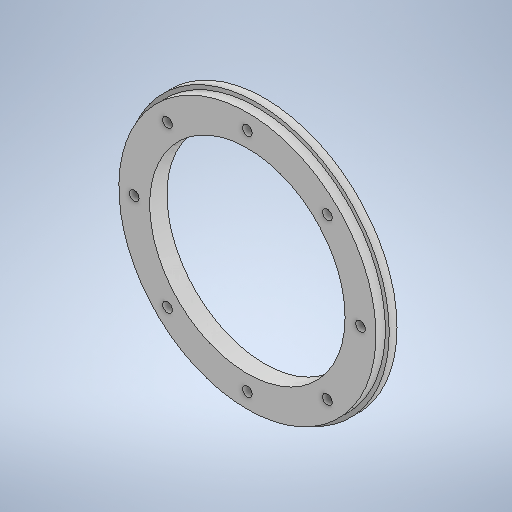
# Autodesk Inventor part: ДМФ 01 31.1 Барабан Опорное кольцо НОС
Saved by Autodesk Inventor 2025 (Build 290162010, 162A)
## iProperties
Created: 2024-04-28
Part Number: ДМФ 01 31.1 Барабан Опорное кольцо НОС
Material: Generic
Document SubType Name: Sheet Metal
Designer: pokla
Density: 1 g/cm^3
Appearance: Default
Stock Number: Опорное_Кольцо_Нос
Sheet Metal Rule: Default
Flat Pattern Width: 33.9 cm
Flat Pattern Length: 33.9 cm
Flat Pattern Area: 1149.21 cm^2
Sheet Metal Width: 339,000 mm
Sheet Metal Length: 339,000 mm
Sheet Metal Area: 114921,000 mm^2
Author: pokla
Autodesk Inventor part; units mm, degrees
ref_plane "YZ Plane" through (0, 0, 0) normal (1, 0, 0) x (0, 1, 0)
ref_plane "XZ Plane" through (0, 0, 0) normal (0, 1, 0) x (-1, 0, 0)
ref_plane "XY Plane" through (0, 0, 0) normal (0, 0, 1) x (1, 0, 0)
sketch "Sketch1" plane through (0, 0, 0) normal (0, 0, 1) x (1, 0, 0)
  circle A0 centre (0, 0) radius 125
  circle A1 centre (0, 0) radius 164.5
  dimension "d0" = 39.5
  dimension "d1" = 250
  constraints: 2 centre point, 1 coincident
  measures "d0" radial gap between concentric circles of A0 A1
  measures "d1" diameter of A0
extrude "Extrusion1" add sketch "Sketch1" along normal blind 41
sketch "Sketch2" plane through (0, 0, 41) normal (0, 0, 1) x (1, 0, 0)
  circle A0 centre (0, 0) radius 164.5 construction
  circle A1 centre (0, 0) radius 125 construction
  line L0 (0, 164.5) -> (0, 125) construction
  circle A2 centre (0, 144.75) radius 6.25
  dimension "d4" = 12.5
  constraints: 3 vertical alignment, 2 end point, 1 centre point, 1 coincident, 1 midpoint, 1 vertical, 2 other
  measures "d4" diameter of A2
extrude "Extrusion2" cut sketch "Sketch2" against normal through all
sketch "Sketch3" plane through (0, 0, 41) normal (0, 0, 1) x (1, 0, 0)
  circle A0 centre (0, 144.75) radius 6.25 projected
  circle A1 centre (0, 144.75) radius 13.75
  point P0 (0, 0)
  dimension "d10" = 27.5
  constraints: 1 centre point
  measures "d10" diameter of A1
extrude "Extrusion3" cut sketch "Sketch3" against normal blind 11
pattern_circular "Circular Pattern1" count 8 over 360 about axis through (0, 0, 0) along (0, 0, 1) of "Extrusion2", "Extrusion3"
sketch "Sketch4" plane through (0, 0, 0) normal (0, 0, -1) x (-1, 0, 0)
  circle A0 centre (0, 0) radius 164.5 projected
  circle A1 centre (0, 0) radius 169.5
  dimension "d13" = 5
  constraints: 1 centre point
  measures "d13" radial gap between concentric circles of A0 A1
extrude "Extrusion4" add sketch "Sketch4" against normal blind 10
sketch "Sketch5" plane through (0, 0, 0) normal (1, 0, 0) x (0, 1, 0)
  line L0 (164.5, 10) -> (-164.5, 10) projected
  line L1 (164.5, 41) -> (-164.5, 41) projected
  line L2 (169.5, 10) -> (-169.5, 10) projected
  line L3 (-169.5, 0) -> (169.5, 0) projected
  line L4 (164.5, 41) -> (164.5, 10)
  line L5 (164.5, 10) -> (164.5, 41) projected
  line L6 (169.5, 10) -> (169.5, 0)
  line L7 (-164.5, 41) -> (-164.5, 10)
  line L8 (-169.5, 10) -> (-169.5, 0)
  line L9 (-164.5, 22) -> (164.5, 22)
  point P0 (0, 0)
  point P1 (164.5, 22)
  dimension "d16" = 19
  dimension "d17" = 41
  constraints: 10 end point, 2 parallel, 2 perpendicular, 2 point on line, 1 collinear
  measures "d16" distance between parallel lines of L1 L9
  measures "d17" distance between parallel lines of L1 L3
extrude "Extrusion5" cut sketch "Sketch5" along normal through all both and the other way through all contours L9 L7 L1 L4
equation "\"d1\" = Вал_ось_диаметр_НОС"
equation "\"BendRadius\" = Thickness"
equation "\"BendReliefWidth\" = Thickness"
equation "\"BendReliefDepth\" = 0.5 * Thickness"
equation "\"CornerReliefSize\" = 4 * Thickness"
equation "\"MinimumRemnant\" = 2 * Thickness"
equation "\"TransitionRadius\" = BendRadius"
equation "\"JacobiRadiusSize\" = BendRadius"
equation "\"GapSize\" = Thickness"
equation "\"Вал_ось_диаметр_НОС\" = 250"
equation "\"Thickness\" = 19"
body "Solid1"
